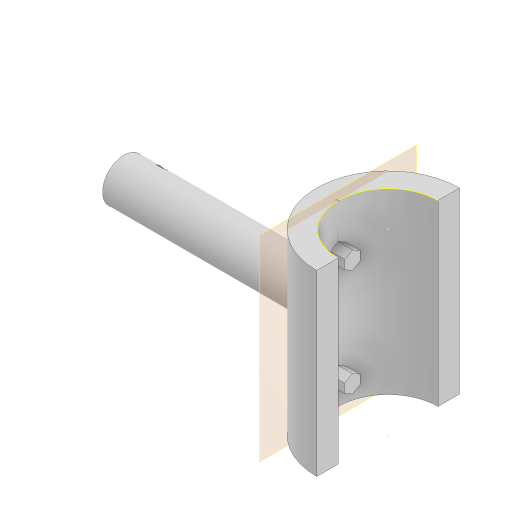
# Autodesk Inventor part: medidor_torque_palanca
Saved by Autodesk Inventor 2024 (Build 280153000, 153)
## iProperties
Created: 2023-05-24
Part Number: medidor_torque_palanca
Material: Generic
Document SubType Name: Modeling
Designer: ferna
Density: 1 g/cm^3
Appearance: Default
Author: ferna
Autodesk Inventor part; units mm, degrees
ref_plane "YZ Plane" through (0, 0, 0) normal (1, 0, 0) x (0, 1, 0)
ref_plane "XZ Plane" through (0, 0, 0) normal (0, 1, 0) x (-1, 0, 0)
ref_plane "XY Plane" through (0, 0, 0) normal (0, 0, 1) x (1, 0, 0)
sketch "Sketch1" plane through (0, 0, 0) normal (0, 1, 0) x (-1, 0, 0)
  circle A0 centre (0, 0) radius 7
  circle A1 centre (0, 0) radius 10
  line L0 (0, 11.563) -> (0, -13.4764)
  point P0 (0, -7)
  point P1 (0, -10)
  point P2 (0, 10)
  point P3 (0, 7)
  dimension "d0" = 14
  dimension "d1" = 20
  constraints: 2 centre point, 2 coincident, 2 end point, 1 vertical
  measures "d0" diameter of A0
  measures "d1" diameter of A1
extrude "Extrusion1" add sketch "Sketch1" along normal blind 25 contours A0 L0 A1 picked at (8.8579, -1.261)
sketch "Sketch2" plane through (0, 25, 0) normal (0, 1, 0) x (1, 0, 0)
  arc A0 (0, 7) -> (0, -7) centre (0, 0) ccw projected
  point P0 (-7, 0)
  constraints: 1 point on circle
ref_plane "Work Plane1" through (-7, 25, 0) normal (1, 0, 0) x (0, 0, -1)
sketch "Sketch3" plane through (-7, 25, 0) normal (1, 0, 0) x (0, 0, -1)
  line L0 (10, 0) -> (-10, 0) projected
  line L1 (0, 0) -> (0, -5)
  line L2 (0, -5) -> (0, -6.25)
  line L3 (0, -5) -> (1.0825, -5.625)
  line L4 (1.0825, -5.625) -> (1.0825, -6.875)
  line L5 (1.0825, -6.875) -> (0, -7.5)
  line L6 (0, -7.5) -> (-1.0825, -6.875)
  line L7 (-1.0825, -6.875) -> (-1.0825, -5.625)
  line L8 (-1.0825, -5.625) -> (0, -5)
  line L9 (0, -6.25) -> (0, -21.25)
  line L10 (0, -21.25) -> (0, -22.5)
  line L11 (0, -22.5) -> (-1.0825, -21.875)
  line L12 (-1.0825, -21.875) -> (-1.0825, -20.625)
  line L13 (-1.0825, -20.625) -> (0, -20)
  line L14 (0, -20) -> (1.0825, -20.625)
  line L15 (1.0825, -20.625) -> (1.0825, -21.875)
  line L16 (1.0825, -21.875) -> (0, -22.5)
  point P0 (0, -25)
  dimension "d4" = 5
  dimension "d5" = 1.25
  dimension "d6" = 15
  dimension "d7" = 1.25
  constraints: 32 end point, 3 vertical, 2 coincident, 1 midpoint, 1 point on line, 26 other
  measures "d4" distance of L1.start L1.end
  measures "d5" distance of L1.end L2.end
  measures "d6" distance of L9.start L9.end
  measures "d7" distance of L9.end L10.end
extrude "Extrusion2" add sketch "Sketch3" along normal blind 2
sketch "Sketch4" plane through (-7, 25, 0) normal (1, 0, 0) x (0, 0, -1)
  line L0 (0, -25) -> (0, 0)
  line L1 (-7, 0) -> (7, 0) projected
  line L2 (0, -12.5) -> (-3, -12.5)
  circle A0 centre (0, -12.5) radius 3
  dimension "d10" = 3
  constraints: 4 end point, 2 midpoint, 1 coincident, 1 horizontal, 1 horizontal alignment, 2 other
  measures "d10" distance of L2.start L2.end
extrude "Extrusion3" add sketch "Sketch4" against normal blind 30
sketch "Sketch5" plane through (0, 0, 0) normal (0, -1, 0) x (1, 0, 0)
  line L0 (-37, 3) -> (-37, -3) projected
  line L1 (-37, -3) -> (-34, -3)
  line L2 (-9.5394, -3) -> (-37, -3) projected
  line L3 (-34, -3) -> (-34, 0)
  line L4 (-34, 0) -> (-34, -1.5)
  line L5 (-34, -1.5) -> (-33, -1.5)
  line L6 (-33, -1.5) -> (-33, -3)
  line L7 (-33, -3) -> (-34.954, -5.8523)
  line L8 (-34.954, -5.8523) -> (-37, -3)
  point P0 (0, 0)
  point P1 (-9.5394, 3)
  dimension "d13" = 3
  dimension "d14" = 1
  constraints: 14 end point, 2 perpendicular, 2 point on line, 1 horizontal, 1 midpoint
  measures "d13" distance of L0.end L1.end
  measures "d14" distance of L4.end L5.end
extrude "Extrusion4" cut sketch "Sketch5" against normal through all
sketch "Sketch6" plane through (0, 0, 0) normal (0, -1, 0) x (1, 0, 0)
  point P0 (0, 0)
body "Solid1"
